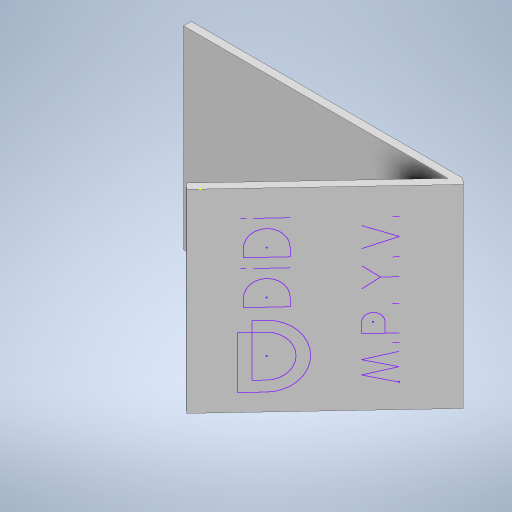
# Autodesk Inventor part: Logo_names
Saved by Autodesk Inventor 2024 (Build 280153000, 153)
## iProperties
Created: 2024-02-25
Part Number: Logo_names
Material: Genérico
Document SubType Name: Modeling
Designer: yovan
Density: 1 g/cm^3
Appearance: Valor por defecto
Author: yovan
Autodesk Inventor part; units mm, degrees
ref_plane "YZ Plane" through (0, 0, 0) normal (1, 0, 0) x (0, 1, 0)
ref_plane "XZ Plane" through (0, 0, 0) normal (0, 1, 0) x (-1, 0, 0)
sketch "Boceto1" plane through (0, 0, 0) normal (0, 0, 1) x (1, 0, 0)
  line L0 (0, 0) -> (350, 0)
  line L1 (350, 0) -> (350, -250)
  line L2 (350, -250) -> (0, -250)
  line L3 (0, -250) -> (0, 0)
  dimension "d0" = 350
  dimension "d1" = 250
  constraints: 8 end point, 2 parallel, 1 horizontal, 1 perpendicular
  measures "d0" distance of L1.end L2.end
  measures "d1" distance of L0.end L1.end
extrude "Extrusión1" add sketch "Boceto1" along normal blind 10
ref_plane "Plano de trabajo1" through (350, -250, 0) normal (-0.7285, 0, -0.685) x (0, 1, 0)
sketch "Boceto2" plane through (350, -250, 0) normal (-0.7285, 0, -0.685) x (0, 1, 0)
  line L0 (0, 0) -> (250, 0) projected
  line L1 (0, 0) -> (250, 0)
  line L2 (250, 0) -> (250, -252)
  line L3 (250, -252) -> (0, -252)
  line L4 (0, -252) -> (0, 0)
  point P0 (250, -239.7606)
  point P1 (250, 0)
  dimension "d5" = 250
  dimension "d6" = 252
  constraints: 8 end point, 2 parallel, 1 horizontal, 1 perpendicular
  measures "d5" distance of L2.end L3.end
  measures "d6" distance of L1.end L2.end
extrude "Extrusión2" add sketch "Boceto2" against normal blind 10
sketch "Boceto3" plane through (357.2851, -250, 6.8503) normal (0.7285, 0, 0.685) x (0.685, 0, -0.7285)
  arc A0 (-179.2335, 22.3949) -> (-179.2335, 102.4229) centre (-179.2335, 62.4089) ccw
  line L0 (-179.2335, 22.3949) -> (-205.9095, 22.3949)
  line L1 (-205.9095, 22.3949) -> (-205.9095, 89.0849)
  line L2 (-179.2335, 89.0849) -> (-192.5715, 89.0849)
  line L3 (-192.5715, 89.0849) -> (-192.5715, 35.7329)
  line L4 (-192.5715, 35.7329) -> (-179.2335, 35.7329)
  arc A1 (-179.2335, 35.7329) -> (-179.2335, 89.0849) centre (-179.2335, 62.4089) ccw
  line L5 (-192.5715, 89.0849) -> (-205.9095, 89.0849)
  line L6 (-192.5715, 102.4229) -> (-192.5715, 89.0849)
  line L7 (-200.5743, 127.8046) -> (-200.5743, 117.1342)
  line L8 (-200.5743, 117.1342) -> (-157.8927, 117.1342)
  line L9 (-157.8927, 117.1342) -> (-157.8927, 127.8046)
  arc A2 (-157.8927, 127.8046) -> (-200.5743, 127.8046) centre (-179.2335, 127.8046) ccw
  line L10 (-200.5743, 160.5789) -> (-203.2419, 160.5789)
  line L11 (-200.5743, 160.5789) -> (-197.9067, 160.5789)
  line L12 (-191.2377, 160.5789) -> (-157.8927, 160.5789)
  line L13 (-200.5743, 183.5325) -> (-200.5743, 172.8621)
  line L14 (-200.5743, 172.8621) -> (-157.8927, 172.8621)
  arc A3 (-157.8927, 183.5325) -> (-200.5743, 183.5325) centre (-179.2335, 183.5325) ccw
  line L15 (-157.8927, 172.8621) -> (-157.8927, 183.5325)
  line L16 (-200.5743, 216.4887) -> (-203.2419, 216.4887)
  line L17 (-200.5743, 216.4887) -> (-197.9067, 216.4887)
  line L18 (-191.2377, 216.4887) -> (-157.8927, 216.4887)
  line L19 (-192.5715, 102.4229) -> (-179.2335, 102.4229)
  line L20 (-75.4492, 148.487) -> (-58.3492, 148.487)
  line L21 (-58.3492, 170.7597) -> (-64.3342, 170.7597)
  line L22 (-92.5492, 135.662) -> (-75.4492, 148.487)
  line L23 (-92.5492, 161.312) -> (-75.4492, 148.487)
  line L24 (-92.5492, 180.5891) -> (-58.3492, 193.4141)
  line L25 (-92.5492, 206.2391) -> (-58.3492, 193.4141)
  line L26 (-58.3492, 215.852) -> (-64.3342, 215.852)
  line L27 (-58.6269, 85.751) -> (-92.8269, 85.751)
  arc A4 (-71.4519, 98.576) -> (-92.8269, 98.576) centre (-82.1394, 98.576) ccw
  line L28 (-71.4519, 98.576) -> (-71.4519, 85.751)
  line L29 (-58.6269, 30.982) -> (-92.8269, 39.532)
  line L30 (-92.8269, 39.532) -> (-58.6269, 48.082)
  line L31 (-92.8269, 56.632) -> (-58.6269, 48.082)
  line L32 (-92.8269, 56.632) -> (-58.6269, 65.182)
  line L33 (-58.6269, 75.322) -> (-64.6119, 75.322)
  line L34 (-92.8269, 85.751) -> (-92.8269, 98.576)
  line L35 (-58.6269, 118.6704) -> (-64.6119, 118.6704)
  point P0 (-239.7606, 250)
  point P1 (-58.6269, 30.982)
  constraints: 72 end point, 10 horizontal, 10 point on circle, 5 centre point, 4 parallel, 4 perpendicular, 2 tangent, 1 point on line, 1 vertical, 1 other
